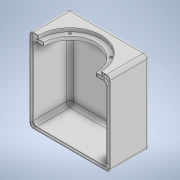
# Autodesk Inventor part: groove
Saved by Autodesk Inventor 2022 (Build 260153000, 153)
## iProperties
Created: 2022-06-28
Part Number: groove
Material: Generic
Document SubType Name: Modeling
Designer: Fuzzyfish
Density: 1 g/cm^3
Appearance: Default
Author: Fuzzyfish
Autodesk Inventor part; units mm, degrees
ref_plane "YZ Plane" through (0, 0, 0) normal (1, 0, 0) x (0, 1, 0)
ref_plane "XZ Plane" through (0, 0, 0) normal (0, 1, 0) x (-1, 0, 0)
sketch "Sketch1" plane through (0, 0, 0) normal (0, 1, 0) x (-1, 0, 0)
  line L0 (0, 0) -> (105, 0)
  line L1 (105, 0) -> (105, -105)
  line L2 (105, -105) -> (0, -105)
  line L3 (0, -105) -> (0, 0)
  circle A0 centre (52.5, -52.5) radius 37.5
  dimension "d0" = 105
  dimension "d1" = 105
  dimension "d2" = 52.5
  dimension "d3" = 52.5
  dimension "d4" = 75
  constraints: 8 end point, 2 parallel, 1 centre point, 1 horizontal, 1 perpendicular
  measures "d0" distance of L0.end L1.end
  measures "d1" distance of L1.end L2.end
  measures "d2" distance from line of L1 A0.centre
  measures "d3" distance from line of L0 A0.centre
  measures "d4" diameter of A0
extrude "Extrusion1" add sketch "Sketch1" along normal blind 5
sketch "Sketch3" plane through (-105, 0, 0) normal (0, 0, 1) x (1, 0, 0)
  line L0 (105, 5) -> (0, 5) projected
  line L1 (0, 5) -> (105, 5)
  line L2 (105, 5) -> (105, -105)
  line L3 (105, -105) -> (0, -105)
  line L4 (0, -105) -> (0, 5)
  line L5 (0, 0) -> (105, 0) projected
  dimension "d7" = 105
  constraints: 8 end point, 2 parallel, 1 horizontal, 1 perpendicular
  measures "d7" distance between parallel lines of L5 L3
extrude "Extrusion2" add sketch "Sketch3" along normal blind 5
sketch "Sketch4" plane through (-105, 0, -105) normal (-1, 0, 0) x (0, 0, 1)
  line L0 (0, 0) -> (0, 5) projected
  line L1 (0, 5) -> (110, 5)
  line L2 (110, 5) -> (110, -105)
  line L3 (110, -105) -> (0, -105)
  line L4 (0, -105) -> (0, 5)
  point P0 (105, 0)
  constraints: 8 end point, 2 parallel, 1 horizontal, 1 perpendicular
extrude "Extrusion3" add sketch "Sketch4" along normal blind 5
sketch "Sketch6" plane through (0, 0, -105) normal (0, 0, -1) x (-1, 0, 0)
  line L0 (0, 5) -> (110, 5) projected
  line L1 (110, -105) -> (110, 5) projected
  line L2 (0, 5) -> (110, 5)
  line L3 (110, 5) -> (110, -105)
  line L4 (110, -105) -> (0, -105)
  line L5 (0, -105) -> (0, 5)
  point P0 (0, 0)
  constraints: 8 end point, 2 parallel, 1 horizontal, 1 perpendicular
extrude "Extrusion4" add sketch "Sketch6" along normal blind 5
sketch "Sketch7" plane through (0, -105, 0) normal (1, 0, 0) x (0, 0, -1)
  line L0 (-5, 0) -> (-5, 110) projected
  line L1 (105, 0) -> (110, 0) projected
  line L2 (-5, 110) -> (110, 110)
  line L3 (110, 110) -> (110, 0)
  line L4 (110, 0) -> (-5, 0)
  line L5 (-5, 0) -> (-5, 110)
  point P0 (0, 105)
  constraints: 8 end point, 2 parallel, 1 horizontal, 1 perpendicular
extrude "Extrusion5" add sketch "Sketch7" along normal blind 5
sketch "Sketch8" plane through (-110, -105, -110) normal (0, -1, 0) x (1, 0, 0)
  line L0 (0, 115) -> (115, 115) projected
  line L1 (0, 0) -> (115, 0) projected
  line L2 (0, 115) -> (115, 115)
  line L3 (115, 115) -> (115, 0)
  line L4 (115, 0) -> (0, 0)
  line L5 (0, 0) -> (0, 115)
  point P0 (110, 110)
  constraints: 8 end point, 2 parallel, 1 horizontal, 1 perpendicular
extrude "Extrusion6" add sketch "Sketch8" along normal blind 5
sketch "Sketch9" plane through (0, 5, 0) normal (0, 1, 0) x (1, 0, 0)
  line L0 (-110, -5) -> (-110, 110) projected
  line L1 (-110, -5) -> (5, -5) projected
  line L2 (5, 110) -> (5, -5) projected
  line L3 (-110, 110) -> (5, 110) projected
  circle A0 centre (-52.5, 52.5) radius 37.5 projected
  line L4 (-110, -5) -> (-110, 110) projected
  line L5 (-110, 110) -> (5, 110) projected
  line L6 (-110, -5) -> (5, -5)
  line L7 (5, -5) -> (5, 110)
  line L8 (5, 110) -> (-110, 110)
  line L9 (-110, 110) -> (-110, -5)
  circle A1 centre (-52.5, 52.5) radius 45
  dimension "d18" = 90
  constraints: 8 end point, 2 parallel, 1 centre point, 1 coincident, 1 horizontal, 1 perpendicular
  measures "d18" diameter of A1
extrude "Extrusion7" add sketch "Sketch9" along normal blind 5 contours L0 L3 L2 L1
sketch "Sketch10" plane through (-52.5, 5, -52.5) normal (0, 1, 0) x (1, 0, 0)
  line L0 (57.5, -57.5) -> (-57.5, -57.5) construction
  line L1 (57.5, 57.5) -> (57.5, -57.5) construction
  line L2 (-57.5, -57.5) -> (57.5, 57.5) construction
  line L3 (57.5, 57.5) -> (-57.5, 57.5) construction
  line L4 (-57.5, 57.5) -> (57.5, -57.5) construction
  circle A0 centre (0, 0) radius 41.75 construction
  circle A1 centre (-29.5217, -29.5217) radius 1.8
  circle A2 centre (-29.5217, 29.5217) radius 1.8
  circle A3 centre (29.5217, 29.5217) radius 1.8
  circle A4 centre (29.5217, -29.5217) radius 1.8
  line L5 (0, -57.5) -> (0, 57.5) construction
  point P0 (52.5, -52.5)
  dimension "d21" = 3.6
  dimension "d22" = 83.5
  dimension "d23" = 3.6
  dimension "d24" = 3.6
  dimension "d25" = 3.6
  dimension "d26" = 45
  constraints: 8 end point, 5 centre point, 4 point on circle, 4 point on line, 3 midpoint, 2 perpendicular
  measures "d21" diameter of A1
  measures "d22" diameter of A0
  measures "d23" diameter of A2
  measures "d24" diameter of A3
  measures "d25" diameter of A4
  measures "d26" angle of L5 L2
extrude "Extrusion8" cut sketch "Sketch10" against normal blind 5
ref_plane "Work Plane1" through (0, 0, -52.5) normal (0, 0, -1) x (-1, 0, 0)
fillet "Fillet2" radius 5 12 edges at (-105, -105, -52.5) (-105, -52.5, -105) (-52.5, -105, -105) (0, -52.5, -105) (0, -52.5, 0) (-52.5, -105, 0) (0, -105, -52.5) (-105, -52.5, 0) (-52.5, 0, -105) (0, 0, -52.5) (-52.5, 0, 0) (-105, 0, -52.5)
fillet "Fillet3" radius 5 12 edges at (-52.5, 10, 5) (-110, 10, -52.5) (-110, -50, 5) (-110, -110, -52.5) (-110, -50, -110) (-52.5, 10, -110) (5, 10, -52.5) (5, -50, 5) (5, -50, -110) (-52.5, -110, -110) (5, -110, -52.5) (-52.5, -110, 5)
sketch "Sketch13" plane through (0, 0, -52.5) normal (0, 0, -1) x (-1, 0, 0)
  arc A0 (5, 0) -> (0, -5) centre (5, -5) ccw projected
  line L0 (0, -5) -> (0, -100) projected
  arc A1 (0, -100) -> (5, -105) centre (5, -100) ccw projected
  line L1 (5, -105) -> (100, -105) projected
  arc A2 (100, -105) -> (105, -100) centre (100, -100) ccw projected
  line L2 (105, -100) -> (105, -5) projected
  arc A3 (105, -5) -> (100, 0) centre (100, -5) ccw projected
  line L3 (100, 0) -> (90, 0) projected
  line L4 (90, 0) -> (90, 5) projected
  line L5 (90, 5) -> (97.5, 5) projected
  line L6 (97.5, 5) -> (97.5, 10) projected
  line L7 (97.5, 10) -> (105, 10) projected
  arc A4 (110, 5) -> (105, 10) centre (105, 5) ccw projected
  line L8 (110, 5) -> (110, -105) projected
  arc A5 (105, -110) -> (110, -105) centre (105, -105) ccw projected
  line L9 (105, -110) -> (0, -110) projected
  arc A6 (-5, -105) -> (0, -110) centre (0, -105) ccw projected
  line L10 (-5, -105) -> (-5, 5) projected
  arc A7 (0, 10) -> (-5, 5) centre (0, 5) ccw projected
  line L11 (0, 10) -> (7.5, 10) projected
  line L12 (7.5, 10) -> (7.5, 5) projected
  line L13 (7.5, 5) -> (15, 5) projected
  line L14 (15, 5) -> (15, 0) projected
  line L15 (15, 0) -> (5, 0) projected
  line L16 (0, -109) -> (105, -109)
  arc A8 (105, -109) -> (109, -105) centre (105, -105) ccw
  line L17 (109, -105) -> (109, 5)
  arc A9 (109, 5) -> (105, 9) centre (105, 5) ccw
  line L18 (105, 9) -> (98.5, 9)
  line L19 (98.5, 9) -> (98.5, 4)
  line L20 (98.5, 4) -> (91, 4)
  line L21 (91, 4) -> (91, 1)
  line L22 (91, 1) -> (100, 1)
  arc A10 (106, -5) -> (100, 1) centre (100, -5) ccw
  line L23 (106, -5) -> (106, -100)
  arc A11 (100, -106) -> (106, -100) centre (100, -100) ccw
  line L24 (100, -106) -> (5, -106)
  arc A12 (-1, -100) -> (5, -106) centre (5, -100) ccw
  line L25 (-1, -100) -> (-1, -5)
  arc A13 (5, 1) -> (-1, -5) centre (5, -5) ccw
  line L26 (5, 1) -> (14, 1)
  line L27 (14, 1) -> (14, 4)
  line L28 (14, 4) -> (6.5, 4)
  line L29 (6.5, 4) -> (6.5, 9)
  line L30 (6.5, 9) -> (0, 9)
  arc A14 (0, 9) -> (-4, 5) centre (0, 5) ccw
  line L31 (-4, 5) -> (-4, -105)
  arc A15 (-4, -105) -> (0, -109) centre (0, -105) ccw
  point P0 (0, 0)
  dimension "d32" = 1
  constraints: 32 end point, 16 point on circle, 8 centre point, 23 other
  measures "d32" distance between parallel lines of L9 L16
split "Split2" plane through (0, 0, -52.5) removes the side toward (0, 0, 1)
extrude "Extrusion10" cut sketch "Sketch13" along normal blind 3 contours A15 L31 A14 L30 L29 L28 L27 L26 A13 L25 A12 L24 A11 L23 A10 L22 L21 L20 L19 L18 A9 L17 A8 L16
equation "\"d2\" = 0.5 * d1"
equation "\"d3\" = 0.5 * d0"
equation "\"d23\" = d21"
equation "\"d24\" = d23"
equation "\"d25\" = d24"
body "Solid1"
